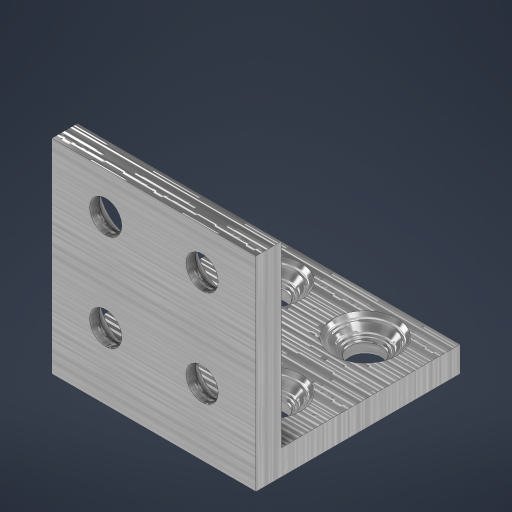
# Autodesk Inventor part: Arashtrix 1in x 1in L-Bracket
Saved by Autodesk Inventor 2024 (Build 280153000, 153)
## iProperties
Created: 2023-10-18
Part Number: Arashtrix 1in x 1in L-Bracket
Material: Generic
Document SubType Name: Modeling
Designer: avsar
Density: 1 g/cm^3
Appearance: Machined 03
Author: avsar
Autodesk Inventor part; units mm, degrees
ref_plane "YZ Plane" through (0, 0, 0) normal (1, 0, 0) x (0, 1, 0)
ref_plane "XZ Plane" through (0, 0, 0) normal (0, 1, 0) x (-1, 0, 0)
ref_plane "XY Plane" through (0, 0, 0) normal (0, 0, 1) x (1, 0, 0)
sketch "Sketch1" plane through (0, 0, 0) normal (1, 0, 0) x (0, 1, 0)
  line L0 (0, 0) -> (25.4, 0)
  line L1 (0, 0) -> (0, -25.4)
  line L2 (0, -25.4) -> (3.175, -25.4)
  line L3 (25.4, 0) -> (25.4, -3.175)
  line L4 (25.4, -3.175) -> (3.175, -3.175)
  line L5 (3.175, -3.175) -> (3.175, -25.4)
  dimension "d0" = 25.4
  dimension "d1" = 25.4
  dimension "d2" = 3.175
  dimension "d3" = 3.175
  constraints: 12 end point, 3 perpendicular, 2 vertical, 1 horizontal
  measures "d0" distance of L0.start L0.end
  measures "d1" distance of L0.start L1.end
  measures "d2" distance of L1.end L2.end
  measures "d3" distance of L0.end L3.end
extrude "Extrusion1" add sketch "Sketch1" along normal mid plane 25.4
sketch "Sketch2" plane through (-12.7, 3.175, -3.175) normal (0, 1, 0) x (1, 0, 0)
  line L0 (0, 0) -> (25.4, 0) construction
  line L1 (25.4, 22.225) -> (25.4, 0) construction
  line L2 (25.4, 22.225) -> (0, 22.225) construction
  line L3 (0, 0) -> (0, 22.225) construction
  line L4 (12.7, 22.225) -> (12.7, 0) construction
  line L5 (0, 11.1125) -> (25.4, 11.1125) construction
  circle A0 centre (18.7, 17.1125) radius 2
  circle A1 centre (6.7, 17.1125) radius 2
  circle A2 centre (6.7, 5.1125) radius 2
  circle A3 centre (18.7, 5.1125) radius 2
  point P0 (12.7, -3.175)
  point P1 (12.7, 11.1125)
  point P2 (12.7, 11.1125)
  dimension "d7" = 4
  dimension "d8" = 6
  dimension "d32" = 6
  dimension "d35" = 360
  constraints: 6 midpoint, 4 centre point, 4 end point, 9 other
  measures "d7" diameter of A0
  measures "d8" horizontal distance of point (12.7, 11.113) A0.centre
  measures "d32" horizontal distance of point (12.7, 11.113) A0.centre
extrude "Extrusion2" cut sketch "Sketch2" against normal through all contours A0
sketch "Sketch3" plane through (12.7, 25.4, -3.175) normal (0, 0, -1) x (-1, 0, 0)
  line L0 (25.4, 0) -> (0, 0) construction
  line L1 (0, -22.225) -> (0, 0) construction
  line L2 (25.4, -22.225) -> (0, -22.225) construction
  line L3 (25.4, 0) -> (25.4, -22.225) construction
  line L4 (12.7, 0) -> (12.7, -22.225) construction
  line L5 (0, -11.1125) -> (25.4, -11.1125) construction
  circle A0 centre (18.7, -5.1125) radius 2
  circle A1 centre (6.7, -5.1125) radius 2
  circle A2 centre (6.7, -17.1125) radius 2
  circle A3 centre (18.7, -17.1125) radius 2
  point P0 (12.7, -25.4)
  point P1 (12.7, -11.1125)
  point P2 (12.7, -11.1125)
  dimension "d13" = 4
  dimension "d14" = 6
  dimension "d39" = 6
  dimension "d42" = 360
  constraints: 6 midpoint, 4 centre point, 4 end point, 9 other
  measures "d13" diameter of A0
  measures "d14" horizontal distance of A0.centre point (12.7, -11.113)
  measures "d39" horizontal distance of point (12.7, -11.113) A0.centre
extrude "Extrusion3" cut sketch "Sketch3" against normal through all contours A0
extrude "Extrusion4" cut sketch "Sketch2" against normal through all contours A1 | A2 | A3
extrude "Extrusion5" cut sketch "Sketch3" against normal through all contours A1 | A2 | A3
hole "Hole3" at (6, 3.175, -8.2875) at (-6, 3.175, -8.2875) at (-6, 3.175, -20.2875) at (6, 3.175, -20.2875) direction (0, -1, 0) diameter 4 end through all countersink diameter 8 countersink angle 90
hole "Hole4" at (6, 8.2875, -3.175) at (-6, 8.2875, -3.175) at (-6, 20.2875, -3.175) at (6, 20.2875, -3.175) direction (0, 0, 1) diameter 4 end through all countersink diameter 8 countersink angle 90
body "Solid1"
